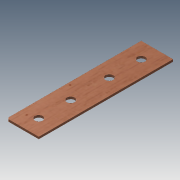
# Autodesk Inventor part: gabarito-suporte-motor-lateral
Saved by Autodesk Inventor 2017 (Build 210142000, 142)
## iProperties
Created: 2018-08-18
Part Number: gabarito-suporte-motor-lateral
Material: Wood (Oak)
Document SubType Name: Sheet Metal
Designer: Luiz Gustavo
Density: 0.76 g/cm^3
Sheet Metal Rule: Default_mm
Appearance: White Oak - Natural Medium Gloss
Author: Luiz Gustavo
Autodesk Inventor part; units mm, degrees
ref_plane "YZ Plane" through (0, 0, 0) normal (1, 0, 0) x (0, 1, 0)
ref_plane "XZ Plane" through (0, 0, 0) normal (0, 1, 0) x (-1, 0, 0)
ref_plane "XY Plane" through (0, 0, 0) normal (0, 0, 1) x (1, 0, 0)
sketch "Sketch1" plane through (0, 0, 0) normal (0, 0, 1) x (1, 0, 0)
  arc A0 (10.4999, 13) -> (8.4999, 15) centre (8.4999, 13) ccw
  arc A1 (-19.5, -109.2599) -> (-17.5, -111.2599) centre (-17.5, -109.2599) ccw
  line L0 (10.4999, 15) -> (-19.5, 15)
  line L1 (-19.5, 15) -> (-19.5, -111.2599)
  line L2 (-19.5, -111.2599) -> (10.4999, -111.2599)
  line L3 (10.4999, -111.2599) -> (10.4999, 15)
  line L4 (-4.5, -111.2599) -> (-4.5, 15) construction
  circle A2 centre (-4.5, 0) radius 3.75
  circle A3 centre (-4.5, -30) radius 3.75
  circle A4 centre (-4.5, -66.2599) radius 3.75
  circle A5 centre (-4.5, -96.2599) radius 3.75
  point P0 (0, 0)
  dimension "d0" = 29.9999
  dimension "d1" = 126.2599
  dimension "d2" = 7.5
  dimension "d3" = 15
  dimension "d4" = 15
  dimension "d5" = 30
  dimension "d6" = 30
  measures "d0" distance of L1.end L2.end
  measures "d1" distance of L2.end L0.start
  measures "d2" diameter of A2
  measures "d3" distance from line of A5.centre L2
  measures "d4" distance from line of L0 A2.centre
  measures "d5" distance of A2.centre A3.centre
  measures "d6" distance of A5.centre A4.centre
extrude "Plate1" add sketch "Sketch1" along normal blind 2 contours L3 L2 A1 L1 L0 A0 | A0 L0 L3
equation "\"d4\" = d3"
equation "\"d6\" = d5"
equation "\"BendRadius\" = Thickness"
equation "\"BendReliefWidth\" = Thickness"
equation "\"BendReliefDepth\" = 0.5 * Thickness"
equation "\"CornerReliefSize\" = 4 * Thickness"
equation "\"MinimumRemnant\" = 2 * Thickness"
equation "\"TransitionRadius\" = BendRadius"
equation "\"JacobiRadiusSize\" = BendRadius"
equation "\"GapSize\" = Thickness"
equation "\"d7\" = BendRadius"
equation "\"Thickness\" = 2"
body "Solid1"
